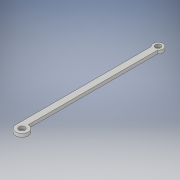
# Autodesk Inventor part: arm
Saved by Autodesk Inventor 2019 (Build 230136000, 136)
## iProperties
Created: 2019-03-31
Part Number: arm
Material: Generic
Document SubType Name: Modeling
Designer: torba
Density: 1 g/cm^3
Appearance: Default
Author: torba
Autodesk Inventor part; units mm, degrees
ref_plane "YZ Plane" through (0, 0, 0) normal (1, 0, 0) x (0, 1, 0)
ref_plane "XZ Plane" through (0, 0, 0) normal (0, 1, 0) x (-1, 0, 0)
ref_plane "XY Plane" through (0, 0, 0) normal (0, 0, 1) x (1, 0, 0)
sketch "Sketch1" plane through (0, 0, 0) normal (0, 1, 0) x (-1, 0, 0)
  arc A0 (5.4989, -12.61) -> (0, -7) centre (0, -12.5) ccw
  arc A1 (-5.669, -4.1064) -> (0, -7) centre (0, 0) ccw
  line L0 (-5.4989, -12.61) -> (-5.669, -4.1064)
  arc A2 (-5.4989, -12.61) -> (5.4989, -12.61) centre (0, -12.5) ccw
  line L1 (5.7488, -0.115) -> (5.4989, -12.61)
  arc A3 (5.7488, -0.115) -> (-5.7488, -0.115) centre (0, 0) ccw
  line L2 (-5.669, -4.1064) -> (-5.7488, -0.115)
  circle A4 centre (0, -12.5) radius 2.5
  circle A5 centre (0, 0) radius 2.75
  circle A6 centre (0, 0) radius 5.75
  dimension "d0" = 7
  dimension "d1" = 5.75
  dimension "d2" = 5.5
  dimension "d3" = 5.5
  dimension "d4" = 5.5
  dimension "d5" = 5
  dimension "d6" = 2.292
  dimension "d7" = 5.75
  dimension "d8" = 5.75
  dimension "d9" = 5.75
  dimension "d10" = 5.75
  dimension "d11" = 5.61
  constraints: 8 point on circle, 7 centre point, 6 end point, 5 tangent, 4 concentric, 1 coincident
  measures "d0" radius of A1
  measures "d1" radius of A3
  measures "d2" diameter of A5
  measures "d3" radius of A2
  measures "d4" radius of A0
  measures "d5" diameter of A4
  measures "d6" angle of L0 L1
  measures "d7" distance from line of point (0, 0) L1
  measures "d8" distance from line of point (0, 0) L0
  measures "d9" distance from line of point (0, 0) L1
  measures "d10" distance from line of point (0, 0) L0
  measures "d11" distance from line of A0.end L1
extrude "Extrusion1" add sketch "Sketch1" along normal blind 3 contours A6 A3
sketch "Sketch3" plane through (0, 3, 0) normal (0, 1, 0) x (1, 0, 0)
  circle A0 centre (0, 0) radius 2.75 projected
  circle A1 centre (0, 0) radius 5.75 projected
  circle A2 centre (0, 0) radius 5.75 projected
  line L0 (-5.75, 0) -> (0, 0) construction
  line L1 (-2.875, 0) -> (-2.875, 127) construction
  line L2 (0, 0) -> (0, 5.75)
  line L3 (-5.75, 127) -> (-5.75, 0)
  arc A3 (-5.75, 0) -> (0, 0) centre (-2.875, 0) ccw
  arc A4 (0, 127) -> (-5.75, 127) centre (-2.875, 127) ccw
  line L4 (0, 5.75) -> (0, 127)
  point P0 (-2.875, 63.5)
  dimension "d18" = 127
  dimension "d19" = 5.75
  constraints: 12 end point, 6 point on circle, 6 tangent, 2 centre point, 2 midpoint, 2 parallel, 1 horizontal, 1 perpendicular
  measures "d18" distance of L1.start L1.end
  measures "d19" diameter of A4
extrude "Extrusion2" add sketch "Sketch3" against normal blind 3 contours L2 A3 A0 | A0 A3 A1 L2 | A1 L3 A4 L4 picked at (-0.9407, -0.3381) picked at (-0.4265, 4.7019)
sketch "Sketch4" plane through (0, 0, 0) normal (0, -1, 0) x (1, 0, 0)
  line L0 (0, -5.75) -> (0, -127) projected
  arc A0 (-5.75, -127) -> (0, -127) centre (-2.875, -127) ccw projected
  line L1 (-5.75, -127) -> (-5.75, 0) projected
  arc A1 (0, -5.75) -> (-5.75, 0) centre (0, 0) ccw projected
  arc A2 (0, 0) -> (-1.3152, 2.4151) centre (-2.875, 0) ccw projected
  line L2 (0, 0) -> (0, -2.75) projected
  arc A3 (0, -2.75) -> (-1.3152, 2.4151) centre (0, 0) ccw projected
  circle A4 centre (0, 0) radius 2.75
  constraints: 1 centre point, 1 coincident, 1 concentric
extrude "Extrusion3" cut sketch "Sketch4" against normal blind 5 contours L2 A4 A2
sketch "Sketch7" plane through (0, 3, 0) normal (0, 1, 0) x (1, 0, 0)
  arc A0 (0, 127) -> (-5.75, 127) centre (-2.875, 127) ccw projected
  circle A1 centre (-2.875, 127) radius 2.5
  circle A2 centre (-2.875, 127) radius 4.5
  point P0 (0, 0)
  dimension "d30" = 5
  dimension "d31" = 9
  constraints: 2 centre point, 2 coincident
  measures "d30" diameter of A1
  measures "d31" diameter of A2
extrude "Extrusion6" add sketch "Sketch7" against normal blind 3
sketch "Sketch8" plane through (0, 3, 0) normal (0, 1, 0) x (1, 0, 0)
  arc A0 (0, 123.5382) -> (-5.75, 123.5382) centre (-2.875, 127) ccw projected
  circle A1 centre (-2.875, 127) radius 2.5
  point P0 (0, 0)
  dimension "d34" = 5
  constraints: 1 centre point, 1 coincident
  measures "d34" diameter of A1
extrude "Extrusion7" cut sketch "Sketch8" against normal blind 3
body "Solid1"
